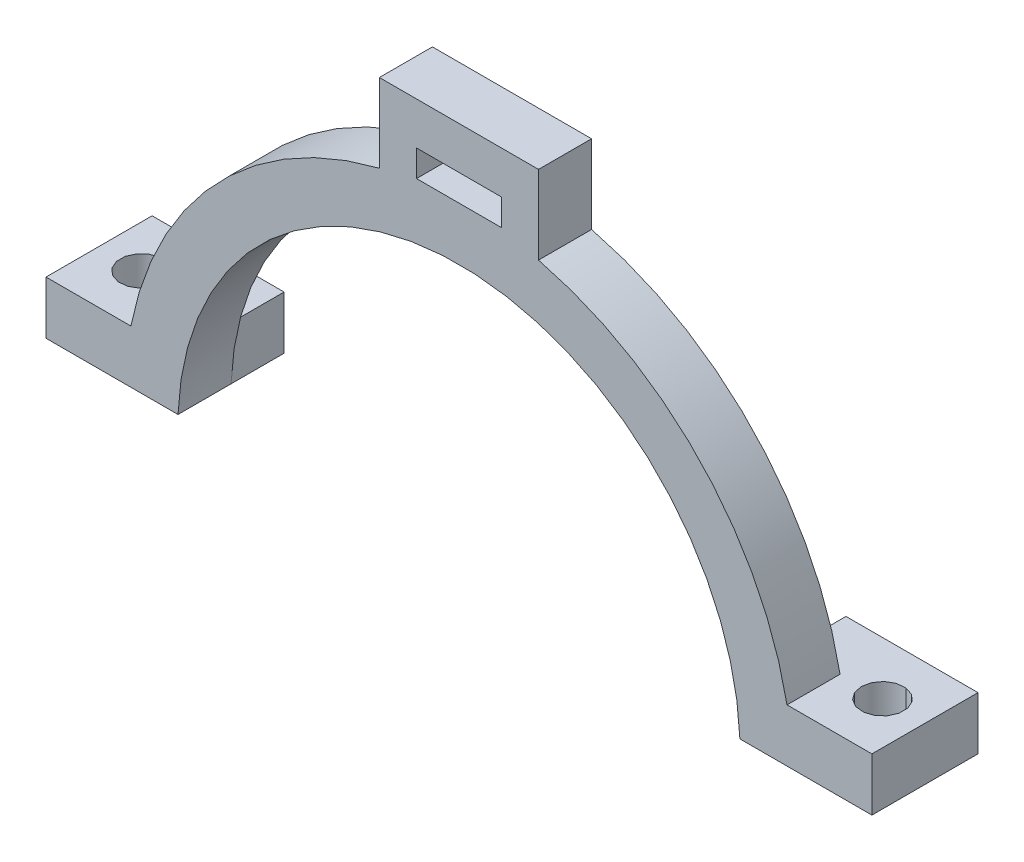
# Autodesk Inventor part: CanBracket
Saved by Autodesk Inventor 2014 SP1 (Build 180222100, 222)
## iProperties
Created: 2017-02-13
Part Number: CanBracket
Material: Generic
Document SubType Name: Modeling
Designer: danielsikar
Density: 1 g/cm^3
Appearance: Default
Author: danielsikar
Autodesk Inventor part; units mm, degrees
ref_plane "YZ Plane" through (0, 0, 0) normal (1, 0, 0) x (0, 1, 0)
ref_plane "Work Plane1" through (0, 0, -3.5) normal (0, 0, 1) x (1, 0, 0)
sketch "Sketch1" plane through (0, 0, -3.5) normal (0, 0, 1) x (1, 0, 0)
  circle A0 centre (0, 0) radius 26.5 projected
  circle A1 centre (0, 0) radius 31.5
  point P0 (0, 0)
  dimension "d1" = 5
  constraints: 1 centre point
  measures "d1" radial gap between concentric circles of A0 A1
extrude "Extrusion1" add sketch "Sketch1" against normal blind 5
sketch "Sketch5" plane through (0, 0, 0) normal (1, 0, 0) x (0, 1, 0)
  line L0 (6.0883, 0) -> (4.0883, 0)
  line L1 (4.0883, 0) -> (4.0883, -15.2563)
  line L2 (4.0883, -15.2563) -> (6.0883, -15.2563)
  line L3 (6.0883, -15.2563) -> (6.0883, 0)
  line L4 (-1, 2.6587) -> (1, 2.6587)
  line L5 (1, 2.6587) -> (1, -12.1151)
  line L6 (1, -12.1151) -> (-1, -12.1151)
  line L7 (-1, -12.1151) -> (-1, 2.6587)
  point P0 (0, 0)
  dimension "d4" = 2
  dimension "d5" = 2
  dimension "d6" = 1
  constraints: 16 end point, 4 parallel, 2 horizontal, 2 perpendicular
  measures "d4" distance of L2.end L1.end
  measures "d5" distance between parallel lines of L5 L7
  measures "d6" distance from line of L7 point (0, 0)
extrude "Extrusion2" cut sketch "Sketch5" along normal through all both and the other way through all contours L4 L5 L6 L7
sketch "Sketch6" plane through (0, 0, -8.5) normal (0, 0, -1) x (-1, 0, 0)
  line L0 (26.4811, 1) -> (31.4841, 1) projected
  line L1 (-31.4841, 1) -> (-26.4811, 1) projected
  arc A0 (26.4811, 1) -> (-26.4811, 1) centre (0, 0) ccw projected
  line L2 (26.4811, 1) -> (31.4841, 1) projected
  arc A1 (31.4841, 1) -> (-31.4841, 1) centre (0, 0) ccw projected
  line L3 (-53.7275, 6) -> (74.5535, 6)
  line L4 (26.4811, 1) -> (30.9233, 1)
  line L5 (30.9233, 1) -> (30.9233, 6)
  line L6 (30.9233, 6) -> (26.4811, 6)
  line L7 (26.4811, 6) -> (26.4811, 1)
  dimension "d9" = 5
  constraints: 10 end point, 3 parallel, 1 horizontal, 1 perpendicular, 1 point on circle, 1 point on line
  measures "d9" distance between parallel lines of L3 L0
extrude "Extrusion3" add sketch "Sketch6" along normal blind 5 contours L7 L3 L5 L0
sketch "Sketch7" plane through (-30.9233, 1, -8.5) normal (-1, 0, 0) x (0, 0, 1)
  line L0 (0, 5) -> (0, 0) projected
  line L1 (0, 5) -> (-5, 5) projected
  line L2 (-5, 0) -> (-5, 5) projected
  line L3 (0, 0) -> (-5, 0) projected
  point P0 (8.5, -1)
extrude "Extrusion4" add sketch "Sketch7" along normal blind 5
sketch "Sketch8" plane through (-35.9233, 6, -8.5) normal (0, 0, 1) x (1, 0, 0)
  arc A0 (5, 0) -> (4.4392, -5) centre (35.9233, -6) ccw projected
  line L0 (5, 0) -> (0, 0) projected
  line L1 (0, -5) -> (0, 0) projected
  line L2 (4.4392, -5) -> (0, -5) projected
extrude "Extrusion5" add sketch "Sketch8" along normal blind 5
sketch "Sketch9" plane through (-35.9233, 1, -8.5) normal (-1, 0, 0) x (0, 0, 1)
  line L0 (-5, 5) -> (5, 5) projected
  line L1 (-5, 5) -> (-5, 0) projected
  line L2 (-5, 0) -> (5, 0) projected
  line L3 (5, 5) -> (5, 0) projected
  point P0 (8.5, -1)
extrude "Extrusion6" add sketch "Sketch9" along normal blind 3
sketch "Sketch10" plane through (-30.9233, 6, -8.5) normal (0, 1, 0) x (1, 0, 0)
  circle A0 centre (-4, 0) radius 2
  point P0 (30.9233, -8.5)
  dimension "d18" = 4
  constraints: 1 centre point
  measures "d18" diameter of A0
extrude "Extrusion7" cut sketch "Sketch10" against normal up to next
mirror "Mirror1" about plane through (0, 0, 0) normal (1, 0, 0) of "Extrusion3", "Extrusion4", "Extrusion5", "Extrusion6", "Extrusion7"
sketch "Sketch11" plane through (0, 0, -8.5) normal (0, 0, -1) x (-1, 0, 0)
  line L0 (31.4841, -1) -> (26.4811, -1) projected
  arc A0 (-26.4811, -1) -> (26.4811, -1) centre (0, 0) ccw projected
  line L1 (-26.4811, -1) -> (-31.4841, -1) projected
  arc A1 (-31.4841, -1) -> (31.4841, -1) centre (0, 0) ccw projected
extrude "Extrusion8" cut sketch "Sketch11" against normal through all
ref_plane "Work Plane2" through (0, 35, 0) normal (0, 1, 0) x (-1, 0, 0)
sketch "Sketch12" plane through (0, 35, 0) normal (0, 1, 0) x (-1, 0, 0)
  line L0 (-30.9233, -3.5) -> (30.9233, -3.5) construction
  line L1 (-30.9233, -8.5) -> (30.9233, -8.5) construction
  line L2 (-7.5, -3.5) -> (7.5, -3.5)
  line L3 (7.5, -3.5) -> (7.5, -8.5)
  line L4 (7.5, -8.5) -> (-7.5, -8.5)
  line L5 (-7.5, -8.5) -> (-7.5, -3.5)
  point P0 (0, 0)
  dimension "d24" = 15
  dimension "d25" = 7.5
  constraints: 8 end point, 2 parallel, 2 point on line, 1 horizontal, 1 perpendicular
  measures "d24" distance of L3.end L4.end
  measures "d25" distance from line of L3 point (0, 0)
extrude "Extrusion9" add sketch "Sketch12" against normal up to next
sketch "Sketch13" plane through (0, 35, 0) normal (0, 1, 0) x (1, 0, 0)
  line L0 (7.5, 3.5) -> (-7.5, 3.5) projected
  line L1 (7.5, 8.5) -> (7.5, 3.5) projected
  line L2 (-7.5, 8.5) -> (7.5, 8.5) projected
  line L3 (-7.5, 3.5) -> (-7.5, 8.5) projected
  point P0 (0, 0)
extrude "Extrusion10" add sketch "Sketch13" along normal blind 3
sketch "Sketch14" plane through (0, 0, -8.5) normal (0, 0, -1) x (-1, 0, 0)
  line L0 (-7.5, 38) -> (7.5, 38) projected
  arc A0 (-7.5, 30.5941) -> (-30.9233, 6) centre (0, 0) ccw projected
  line L1 (-4, 34) -> (4, 34)
  line L2 (4, 34) -> (4, 31.5)
  line L3 (4, 31.5) -> (-4, 31.5)
  line L4 (-4, 31.5) -> (-4, 34)
  dimension "d30" = 8
  dimension "d31" = 2.5
  dimension "d32" = 4
  dimension "d33" = 4
  constraints: 8 end point, 2 parallel, 1 horizontal, 1 perpendicular
  measures "d30" distance of L2.end L3.end
  measures "d31" distance of L1.end L2.end
  measures "d32" distance from line of L2 A0.centre
  measures "d33" distance between parallel lines of L1 L0
extrude "Extrusion11" cut sketch "Sketch14" against normal blind 5
body "Solid1"
